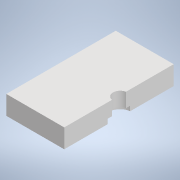
# Autodesk Inventor part: 15_Base_Dietro
Saved by Autodesk Inventor 2020 (Build 240168000, 168)
## iProperties
Created: 2019-10-17
Part Number: 15_Base_Dietro
Material: Generico
Document SubType Name: Modeling
Designer: socci
Density: 1 g/cm^3
Appearance: Default
Author: socci
Autodesk Inventor part; units mm, degrees
ref_plane "YZ Plane" through (0, 0, 0) normal (1, 0, 0) x (0, 1, 0)
ref_plane "XZ Plane" through (0, 0, 0) normal (0, 1, 0) x (-1, 0, 0)
ref_plane "XY Plane" through (0, 0, 0) normal (0, 0, 1) x (1, 0, 0)
sketch "Schizzo1" plane through (0, 0, 0) normal (0, 1, 0) x (-1, 0, 0)
  line L0 (9.5, 50) -> (-9.5, 50)
  line L1 (-9.5, 50) -> (-9.5, -50)
  line L2 (-9.5, -50) -> (9.5, -50)
  line L3 (9.5, -50) -> (9.5, 50)
  line L4 (9.5, 50) -> (-9.5, -50) construction
  line L5 (-9.5, 50) -> (9.5, -50) construction
  point P0 (0, 0)
  point P1 (0, 0)
  point P2 (0, 0)
  dimension "d0" = 19
  dimension "d15" = 100
  constraints: 12 end point, 3 midpoint, 2 parallel, 1 coincident, 1 horizontal, 1 perpendicular
  measures "d0" distance of L0.start L0.end
  measures "d15" distance of L2.end L0.start
extrude "Estrusione1" add sketch "Schizzo1" along normal blind 16
sketch "Schizzo2" plane through (0, 0, 0) normal (0, -1, 0) x (1, 0, 0)
  line L0 (9.5, 50) -> (9.5, -50) projected
  line L1 (9.5, 0) -> (10.5, 0)
  line L2 (9.5, 0) -> (10.5, 0) construction
  circle A0 centre (10.5, 0) radius 9.5
  point P0 (0, 0)
  dimension "d9" = 1
  dimension "d10" = 0
  dimension "d11" = 19
  constraints: 4 end point, 2 horizontal, 1 centre point, 1 coincident, 1 collinear, 1 midpoint
  measures "d9" distance of L1.start L1.end
  measures "d10" distance between parallel lines of L1 L2
  measures "d11" diameter of A0
extrude "Estrusione2" cut sketch "Schizzo2" against normal blind 4
sketch "Schizzo4" plane through (0, 4, 0) normal (0, -1, 0) x (1, 0, 0)
  line L0 (9.5, 9.4472) -> (9.5, -9.4472) projected
  line L1 (9.5, 0) -> (10.5, 0)
  line L2 (9.5, 0) -> (10.5, 0) construction
  circle A0 centre (10.5, 0) radius 6
  point P0 (0, 0)
  point P1 (24.5, 9.5)
  point P2 (24.5, -9.5)
  point P3 (9.5, -9.4472)
  dimension "d12" = 1
  dimension "d13" = 0
  dimension "d14" = 12
  constraints: 4 end point, 2 horizontal, 1 centre point, 1 coincident, 1 collinear, 2 other
  measures "d12" distance of L1.start L1.end
  measures "d13" distance between parallel lines of L1 L2
  measures "d14" diameter of A0
extrude "Estrusione3" cut sketch "Schizzo4" against normal blind 26
sketch "Schizzo8" plane through (0, 16, 0) normal (0, 1, 0) x (1, 0, 0)
  arc A0 (9.5, 5.9161) -> (9.5, -5.9161) centre (10.5, 0) ccw projected
  circle A1 centre (10.5, 0) radius 20
  line L0 (-9.5, 50) -> (-9.5, -50) projected
  line L1 (-9.5, 0) -> (-9.5, -50)
  line L2 (-9.5, -50) -> (0, -50)
  line L3 (-9.5, -50) -> (9.5, -50) projected
  line L4 (0, -50) -> (0, -17.022)
  line L5 (9.5, 50) -> (-9.5, 50) projected
  line L6 (-9.5, 0) -> (-9.5, 50)
  line L7 (-9.5, 50) -> (0, 50)
  line L8 (0, 50) -> (0, 17.022)
  point P0 (0, 0)
  dimension "d17" = 40
  constraints: 12 end point, 4 vertical, 3 point on circle, 2 midpoint, 1 centre point, 1 coincident
  measures "d17" diameter of A1
extrude "Estrusione4" cut sketch "Schizzo8" against normal blind 16 contours A1 L0 L5 L8 | L4 L2 L0 A1
